Autodesk Fusion 360 part; units mm, degrees
(part 2 of 5)
  spline S13 degree 5 poles (-172.8984, -52.5106) (-172.8973, -52.5173) (-172.8952, -52.5307) (-172.8927, -52.5509) (-172.8903, -52.5779) (-172.8889, -52.6119) (-172.8884, -52.6459) (-172.8887, -52.6801) (-172.8892, -52.7143) (-172.89, -52.7486) (-172.8911, -52.7829) (-172.8924, -52.8172) (-172.8943, -52.8516) (-172.8966, -52.886) (-172.8994, -52.9205) (-172.9027, -52.955) (-172.9064, -52.9895) (-172.9104, -53.0241) (-172.9148, -53.0587) (-172.9194, -53.0933) (-172.9243, -53.1279) (-172.9295, -53.1625) (-172.9351, -53.1972) (-172.9409, -53.2319) (-172.9471, -53.2666) (-172.9535, -53.3013) (-172.9603, -53.336) (-172.9673, -53.3707) (-172.9746, -53.4054) (-172.9822, -53.4402) (-172.99, -53.4749) (-172.9981, -53.5097) (-173.0064, -53.5444) (-173.015, -53.5792) (-173.0239, -53.614) (-173.033, -53.6487) (-173.0424, -53.6835) (-173.052, -53.7183) (-173.0618, -53.753) (-173.0719, -53.7878) (-173.0822, -53.8225) (-173.0928, -53.8573) (-173.1036, -53.892) (-173.1146, -53.9267) (-173.1259, -53.9615) (-173.1373, -53.9962) (-173.1491, -54.0309) (-173.161, -54.0656) (-173.1731, -54.1003) (-173.1855, -54.135) (-173.1981, -54.1696) (-173.2109, -54.2043) (-173.2239, -54.2389) (-173.2371, -54.2735) (-173.2506, -54.3081) (-173.2642, -54.3427) (-173.2781, -54.3773) (-173.2921, -54.4118) (-173.3064, -54.4464) (-173.3209, -54.4809) (-173.3356, -54.5154) (-173.3504, -54.5499) (-173.3655, -54.5843) (-173.3808, -54.6188) (-173.3963, -54.6532) (-173.412, -54.6875) (-173.4278, -54.7219) (-173.4439, -54.7562) (-173.4602, -54.7906) (-173.4766, -54.8248) (-173.4933, -54.8591) (-173.5068, -54.8865) (-173.517, -54.907) (-173.5238, -54.9207) (-173.5272, -54.9275) knots 0 0 0 0 0 0 0.01428571 0.02857143 0.04285714 0.05714286 0.07142857 0.08571429 0.1 0.11428571 0.12857143 0.14285714 0.15714286 0.17142857 0.18571429 0.2 0.21428571 0.22857143 0.24285714 0.25714286 0.27142857 0.28571429 0.3 0.31428571 0.32857143 0.34285714 0.35714286 0.37142857 0.38571429 0.4 0.41428571 0.42857143 0.44285714 0.45714286 0.47142857 0.48571429 0.5 0.51428571 0.52857143 0.54285714 0.55714286 0.57142857 0.58571429 0.6 0.61428571 0.62857143 0.64285714 0.65714286 0.67142857 0.68571429 0.7 0.71428571 0.72857143 0.74285714 0.75714286 0.77142857 0.78571429 0.8 0.81428571 0.82857143 0.84285714 0.85714286 0.87142857 0.88571429 0.9 0.91428571 0.92857143 0.94285714 0.95714286 0.97142857 0.98571429 1 1 1 1 1 1
  line L13 (-172.8984, -52.5106) -> (-172.9699, -52.085)
  arc A26 (-172.5797, -51.5128) -> (-172.9699, -52.085) centre (-172.4768, -52.0021) ccw
  arc A27 (-172.5797, -51.5128) -> (-171.7948, -51.3195) centre (-175, -40) ccw
  arc A28 (-171.1835, -51.6448) -> (-171.7948, -51.3195) centre (-171.6586, -51.8006) ccw
  line L14 (-171.1835, -51.6448) -> (-171.0491, -52.0549)
  spline S14 degree 5 poles (-171.0491, -52.0549) (-171.047, -52.0614) (-171.0426, -52.0742) (-171.0354, -52.0933) (-171.025, -52.1183) (-171.0105, -52.1491) (-170.995, -52.1794) (-170.979, -52.2096) (-170.9626, -52.2396) (-170.9459, -52.2696) (-170.9291, -52.2995) (-170.9119, -52.3292) (-170.8943, -52.3588) (-170.8763, -52.3882) (-170.8578, -52.4175) (-170.8388, -52.4465) (-170.8195, -52.4753) (-170.7999, -52.5041) (-170.78, -52.5327) (-170.7598, -52.5612) (-170.7393, -52.5895) (-170.7186, -52.6178) (-170.6977, -52.6459) (-170.6764, -52.6739) (-170.6548, -52.7018) (-170.633, -52.7295) (-170.6109, -52.7571) (-170.5885, -52.7846) (-170.5659, -52.812) (-170.543, -52.8392) (-170.52, -52.8664) (-170.4967, -52.8934) (-170.4731, -52.9203) (-170.4494, -52.9471) (-170.4254, -52.9737) (-170.4011, -53.0003) (-170.3767, -53.0267) (-170.352, -53.053) (-170.3272, -53.0792) (-170.3021, -53.1053) (-170.2768, -53.1313) (-170.2513, -53.1572) (-170.2256, -53.1829) (-170.1997, -53.2086) (-170.1736, -53.2341) (-170.1473, -53.2595) (-170.1208, -53.2848) (-170.0942, -53.31) (-170.0673, -53.3351) (-170.0402, -53.36) (-170.013, -53.3849) (-169.9856, -53.4096) (-169.9579, -53.4342) (-169.9301, -53.4588) (-169.9022, -53.4832) (-169.874, -53.5074) (-169.8457, -53.5316) (-169.8172, -53.5557) (-169.7885, -53.5796) (-169.7596, -53.6035) (-169.7306, -53.6272) (-169.7014, -53.6508) (-169.6721, -53.6743) (-169.6425, -53.6977) (-169.6128, -53.721) (-169.583, -53.7442) (-169.553, -53.7672) (-169.5228, -53.7901) (-169.4924, -53.813) (-169.4619, -53.8357) (-169.4313, -53.8583) (-169.4066, -53.8763) (-169.388, -53.8897) (-169.3756, -53.8986) (-169.3694, -53.9031) knots 0 0 0 0 0 0 0.01428571 0.02857143 0.04285714 0.05714286 0.07142857 0.08571429 0.1 0.11428571 0.12857143 0.14285714 0.15714286 0.17142857 0.18571429 0.2 0.21428571 0.22857143 0.24285714 0.25714286 0.27142857 0.28571429 0.3 0.31428571 0.32857143 0.34285714 0.35714286 0.37142857 0.38571429 0.4 0.41428571 0.42857143 0.44285714 0.45714286 0.47142857 0.48571429 0.5 0.51428571 0.52857143 0.54285714 0.55714286 0.57142857 0.58571429 0.6 0.61428571 0.62857143 0.64285714 0.65714286 0.67142857 0.68571429 0.7 0.71428571 0.72857143 0.74285714 0.75714286 0.77142857 0.78571429 0.8 0.81428571 0.82857143 0.84285714 0.85714286 0.87142857 0.88571429 0.9 0.91428571 0.92857143 0.94285714 0.95714286 0.97142857 0.98571429 1 1 1 1 1 1
  arc A29 (-169.3694, -53.9031) -> (-168.5105, -53.5236) centre (-175, -40) ccw
  spline S15 degree 5 poles (-168.7463, -51.0373) (-168.7429, -51.0432) (-168.7364, -51.0551) (-168.7271, -51.0732) (-168.7157, -51.0978) (-168.7027, -51.1292) (-168.6906, -51.1611) (-168.6791, -51.1933) (-168.668, -51.2256) (-168.657, -51.2581) (-168.6463, -51.2907) (-168.6358, -51.3234) (-168.6257, -51.3563) (-168.6161, -51.3895) (-168.607, -51.4228) (-168.5983, -51.4564) (-168.59, -51.4901) (-168.582, -51.524) (-168.5742, -51.5579) (-168.5667, -51.592) (-168.5595, -51.6263) (-168.5526, -51.6606) (-168.5459, -51.695) (-168.5395, -51.7296) (-168.5334, -51.7643) (-168.5276, -51.7992) (-168.5221, -51.8341) (-168.5168, -51.8691) (-168.5118, -51.9043) (-168.507, -51.9395) (-168.5025, -51.9748) (-168.4982, -52.0103) (-168.4942, -52.0458) (-168.4904, -52.0814) (-168.4868, -52.1171) (-168.4835, -52.1529) (-168.4804, -52.1887) (-168.4775, -52.2247) (-168.4749, -52.2607) (-168.4725, -52.2968) (-168.4703, -52.333) (-168.4684, -52.3693) (-168.4666, -52.4056) (-168.4651, -52.442) (-168.4638, -52.4785) (-168.4627, -52.5151) (-168.4618, -52.5517) (-168.4612, -52.5884) (-168.4607, -52.6251) (-168.4605, -52.6619) (-168.4604, -52.6988) (-168.4606, -52.7357) (-168.461, -52.7727) (-168.4616, -52.8098) (-168.4624, -52.8469) (-168.4634, -52.8841) (-168.4646, -52.9213) (-168.466, -52.9586) (-168.4676, -52.9959) (-168.4694, -53.0333) (-168.4714, -53.0707) (-168.4736, -53.1082) (-168.476, -53.1458) (-168.4785, -53.1833) (-168.4813, -53.221) (-168.4843, -53.2586) (-168.4875, -53.2964) (-168.4908, -53.3341) (-168.4944, -53.3719) (-168.4981, -53.4098) (-168.5021, -53.4477) (-168.5053, -53.478) (-168.5079, -53.5008) (-168.5097, -53.516) (-168.5105, -53.5236) knots 0 0 0 0 0 0 0.01428571 0.02857143 0.04285714 0.05714286 0.07142857 0.08571429 0.1 0.11428571 0.12857143 0.14285714 0.15714286 0.17142857 0.18571429 0.2 0.21428571 0.22857143 0.24285714 0.25714286 0.27142857 0.28571429 0.3 0.31428571 0.32857143 0.34285714 0.35714286 0.37142857 0.38571429 0.4 0.41428571 0.42857143 0.44285714 0.45714286 0.47142857 0.48571429 0.5 0.51428571 0.52857143 0.54285714 0.55714286 0.57142857 0.58571429 0.6 0.61428571 0.62857143 0.64285714 0.65714286 0.67142857 0.68571429 0.7 0.71428571 0.72857143 0.74285714 0.75714286 0.77142857 0.78571429 0.8 0.81428571 0.82857143 0.84285714 0.85714286 0.87142857 0.88571429 0.9 0.91428571 0.92857143 0.94285714 0.95714286 0.97142857 0.98571429 1 1 1 1 1 1
  line L15 (-168.7463, -51.0373) -> (-168.959, -50.6618)
  arc A30 (-168.788, -49.9907) -> (-168.959, -50.6618) centre (-168.524, -50.4153) ccw
  arc A31 (-168.788, -49.9907) -> (-168.1167, -49.5406) centre (-175, -40) ccw
  arc A32 (-167.4309, -49.6372) -> (-168.1167, -49.5406) centre (-167.8241, -49.9461) ccw
  line L16 (-167.4309, -49.6372) -> (-167.1643, -49.9766)
  spline S16 degree 5 poles (-167.1643, -49.9766) (-167.1601, -49.982) (-167.1516, -49.9925) (-167.1384, -50.008) (-167.12, -50.0279) (-167.0959, -50.0519) (-167.0709, -50.0752) (-167.0455, -50.098) (-167.0199, -50.1206) (-166.994, -50.1431) (-166.9679, -50.1654) (-166.9416, -50.1875) (-166.915, -50.2093) (-166.888, -50.2308) (-166.8606, -50.2519) (-166.8329, -50.2727) (-166.8048, -50.2932) (-166.7765, -50.3134) (-166.748, -50.3335) (-166.7193, -50.3534) (-166.6904, -50.3731) (-166.6613, -50.3925) (-166.632, -50.4118) (-166.6024, -50.4308) (-166.5726, -50.4496) (-166.5426, -50.4682) (-166.5124, -50.4866) (-166.4819, -50.5048) (-166.4513, -50.5228) (-166.4206, -50.5406) (-166.3896, -50.5582) (-166.3585, -50.5756) (-166.3271, -50.5928) (-166.2956, -50.6099) (-166.264, -50.6267) (-166.2321, -50.6434) (-166.2001, -50.6599) (-166.1679, -50.6762) (-166.1356, -50.6923) (-166.1031, -50.7082) (-166.0705, -50.724) (-166.0377, -50.7396) (-166.0047, -50.755) (-165.9716, -50.7702) (-165.9384, -50.7853) (-165.905, -50.8001) (-165.8714, -50.8149) (-165.8377, -50.8294) (-165.8039, -50.8438) (-165.7699, -50.858) (-165.7358, -50.872) (-165.7016, -50.8859) (-165.6672, -50.8996) (-165.6327, -50.9131) (-165.5981, -50.9265) (-165.5633, -50.9397) (-165.5284, -50.9527) (-165.4934, -50.9655) (-165.4583, -50.9782) (-165.423, -50.9908) (-165.3876, -51.0031) (-165.3521, -51.0153) (-165.3165, -51.0274) (-165.2807, -51.0393) (-165.2449, -51.051) (-165.2089, -51.0625) (-165.1728, -51.0739) (-165.1366, -51.0852) (-165.1003, -51.0962) (-165.0638, -51.1072) (-165.0273, -51.1179) (-164.998, -51.1264) (-164.9759, -51.1327) (-164.9612, -51.1368) (-164.9538, -51.1389) knots 0 0 0 0 0 0 0.01428571 0.02857143 0.04285714 0.05714286 0.07142857 0.08571429 0.1 0.11428571 0.12857143 0.14285714 0.15714286 0.17142857 0.18571429 0.2 0.21428571 0.22857143 0.24285714 0.25714286 0.27142857 0.28571429 0.3 0.31428571 0.32857143 0.34285714 0.35714286 0.37142857 0.38571429 0.4 0.41428571 0.42857143 0.44285714 0.45714286 0.47142857 0.48571429 0.5 0.51428571 0.52857143 0.54285714 0.55714286 0.57142857 0.58571429 0.6 0.61428571 0.62857143 0.64285714 0.65714286 0.67142857 0.68571429 0.7 0.71428571 0.72857143 0.74285714 0.75714286 0.77142857 0.78571429 0.8 0.81428571 0.82857143 0.84285714 0.85714286 0.87142857 0.88571429 0.9 0.91428571 0.92857143 0.94285714 0.95714286 0.97142857 0.98571429 1 1 1 1 1 1
  arc A33 (-164.9538, -51.1389) -> (-164.2766, -50.4885) centre (-175, -40) ccw
  spline S17 degree 5 poles (-165.3485, -48.2328) (-165.3433, -48.2372) (-165.3331, -48.2461) (-165.3182, -48.26) (-165.299, -48.2792) (-165.276, -48.3042) (-165.2538, -48.3301) (-165.232, -48.3564) (-165.2104, -48.383) (-165.189, -48.4097) (-165.1678, -48.4367) (-165.1468, -48.4638) (-165.1261, -48.4913) (-165.1057, -48.5192) (-165.0857, -48.5474) (-165.0661, -48.576) (-165.0467, -48.6048) (-165.0276, -48.6339) (-165.0087, -48.6632) (-164.99, -48.6927) (-164.9715, -48.7223) (-164.9532, -48.7522) (-164.9352, -48.7823) (-164.9174, -48.8126) (-164.8998, -48.8432) (-164.8824, -48.8739) (-164.8653, -48.9048) (-164.8483, -48.936) (-164.8316, -48.9673) (-164.8151, -48.9987) (-164.7987, -49.0304) (-164.7826, -49.0622) (-164.7666, -49.0942) (-164.7509, -49.1264) (-164.7353, -49.1587) (-164.72, -49.1912) (-164.7048, -49.2238) (-164.6898, -49.2566) (-164.675, -49.2896) (-164.6604, -49.3227) (-164.646, -49.356) (-164.6317, -49.3894) (-164.6177, -49.4229) (-164.6038, -49.4566) (-164.5901, -49.4904) (-164.5765, -49.5244) (-164.5632, -49.5585) (-164.55, -49.5928) (-164.537, -49.6272) (-164.5242, -49.6617) (-164.5116, -49.6963) (-164.4991, -49.7311) (-164.4868, -49.766) (-164.4747, -49.801) (-164.4628, -49.8361) (-164.451, -49.8714) (-164.4394, -49.9068) (-164.4279, -49.9423) (-164.4167, -49.9779) (-164.4056, -50.0137) (-164.3946, -50.0495) (-164.3839, -50.0855) (-164.3733, -50.1216) (-164.3629, -50.1578) (-164.3526, -50.1941) (-164.3425, -50.2305) (-164.3326, -50.2671) (-164.3228, -50.3037) (-164.3132, -50.3404) (-164.3038, -50.3773) (-164.2946, -50.4142) (-164.2873, -50.4439) (-164.2819, -50.4662) (-164.2783, -50.481) (-164.2766, -50.4885) knots 0 0 0 0 0 0 0.01428571 0.02857143 0.04285714 0.05714286 0.07142857 0.08571429 0.1 0.11428571 0.12857143 0.14285714 0.15714286 0.17142857 0.18571429 0.2 0.21428571 0.22857143 0.24285714 0.25714286 0.27142857 0.28571429 0.3 0.31428571 0.32857143 0.34285714 0.35714286 0.37142857 0.38571429 0.4 0.41428571 0.42857143 0.44285714 0.45714286 0.47142857 0.48571429 0.5 0.51428571 0.52857143 0.54285714 0.55714286 0.57142857 0.58571429 0.6 0.61428571 0.62857143 0.64285714 0.65714286 0.67142857 0.68571429 0.7 0.71428571 0.72857143 0.74285714 0.75714286 0.77142857 0.78571429 0.8 0.81428571 0.82857143 0.84285714 0.85714286 0.87142857 0.88571429 0.9 0.91428571 0.92857143 0.94285714 0.95714286 0.97142857 0.98571429 1 1 1 1 1 1
  line L17 (-165.3485, -48.2328) -> (-165.6768, -47.9527)
  arc A34 (-165.7456, -47.2636) -> (-165.6768, -47.9527) centre (-165.3523, -47.5723) ccw
  arc A35 (-165.7456, -47.2636) -> (-165.2687, -46.611) centre (-175, -40) ccw
  arc A36 (-164.5912, -46.4673) -> (-165.2687, -46.611) centre (-164.8551, -46.892) ccw
  line L18 (-164.5912, -46.4673) -> (-164.2247, -46.695)
  spline S18 degree 5 poles (-164.2247, -46.695) (-164.2189, -46.6986) (-164.2073, -46.7056) (-164.1896, -46.7156) (-164.1654, -46.728) (-164.1346, -46.7423) (-164.1032, -46.7557) (-164.0715, -46.7684) (-164.0397, -46.7809) (-164.0077, -46.7932) (-163.9755, -46.8052) (-163.9433, -46.817) (-163.9108, -46.8284) (-163.8781, -46.8393) (-163.8451, -46.8498) (-163.8119, -46.8598) (-163.7786, -46.8695) (-163.7451, -46.8789) (-163.7114, -46.888) (-163.6776, -46.8969) (-163.6437, -46.9055) (-163.6097, -46.9138) (-163.5756, -46.9219) (-163.5413, -46.9296) (-163.5068, -46.9371) (-163.4723, -46.9443) (-163.4376, -46.9512) (-163.4028, -46.9579) (-163.3679, -46.9644) (-163.3329, -46.9705) (-163.2978, -46.9765) (-163.2625, -46.9822) (-163.2272, -46.9877) (-163.1918, -46.9929) (-163.1563, -46.9979) (-163.1207, -47.0027) (-163.0849, -47.0073) (-163.0491, -47.0116) (-163.0132, -47.0156) (-162.9772, -47.0195) (-162.9412, -47.0232) (-162.905, -47.0266) (-162.8688, -47.0298) (-162.8325, -47.0328) (-162.7961, -47.0356) (-162.7596, -47.0381) (-162.723, -47.0405) (-162.6864, -47.0426) (-162.6497, -47.0446) (-162.6129, -47.0463) (-162.5761, -47.0478) (-162.5392, -47.0491) (-162.5022, -47.0503) (-162.4651, -47.0512) (-162.428, -47.0519) (-162.3909, -47.0524) (-162.3536, -47.0527) (-162.3163, -47.0528) (-162.2789, -47.0527) (-162.2415, -47.0524) (-162.204, -47.0519) (-162.1665, -47.0513) (-162.1289, -47.0504) (-162.0912, -47.0493) (-162.0535, -47.0481) (-162.0157, -47.0466) (-161.9779, -47.045) (-161.9401, -47.0432) (-161.9021, -47.0411) (-161.8642, -47.0389) (-161.8262, -47.0365) (-161.7957, -47.0345) (-161.7729, -47.0328) (-161.7576, -47.0317) (-161.75, -47.0311) knots 0 0 0 0 0 0 0.01428571 0.02857143 0.04285714 0.05714286 0.07142857 0.08571429 0.1 0.11428571 0.12857143 0.14285714 0.15714286 0.17142857 0.18571429 0.2 0.21428571 0.22857143 0.24285714 0.25714286 0.27142857 0.28571429 0.3 0.31428571 0.32857143 0.34285714 0.35714286 0.37142857 0.38571429 0.4 0.41428571 0.42857143 0.44285714 0.45714286 0.47142857 0.48571429 0.5 0.51428571 0.52857143 0.54285714 0.55714286 0.57142857 0.58571429 0.6 0.61428571 0.62857143 0.64285714 0.65714286 0.67142857 0.68571429 0.7 0.71428571 0.72857143 0.74285714 0.75714286 0.77142857 0.78571429 0.8 0.81428571 0.82857143 0.84285714 0.85714286 0.87142857 0.88571429 0.9 0.91428571 0.92857143 0.94285714 0.95714286 0.97142857 0.98571429 1 1 1 1 1 1
  arc A37 (-161.75, -47.0311) -> (-161.336, -46.1883) centre (-175, -40) ccw
  spline S19 degree 5 poles (-163.1147, -44.4353) (-163.1084, -44.4376) (-163.0957, -44.4425) (-163.077, -44.4504) (-163.0524, -44.4619) (-163.0222, -44.4776) (-162.9925, -44.4943) (-162.963, -44.5116) (-162.9337, -44.5292) (-162.9044, -44.547) (-162.8752, -44.5651) (-162.8462, -44.5834) (-162.8173, -44.6022) (-162.7887, -44.6214) (-162.7602, -44.6411) (-162.732, -44.6612) (-162.704, -44.6816) (-162.676, -44.7024) (-162.6483, -44.7235) (-162.6206, -44.7448) (-162.5931, -44.7664) (-162.5657, -44.7882) (-162.5384, -44.8103) (-162.5113, -44.8327) (-162.4844, -44.8554) (-162.4575, -44.8783) (-162.4308, -44.9015) (-162.4043, -44.925) (-162.3778, -44.9487) (-162.3515, -44.9726) (-162.3254, -44.9968) (-162.2993, -45.0211) (-162.2734, -45.0457) (-162.2476, -45.0706) (-162.2219, -45.0956) (-162.1964, -45.1209) (-162.1709, -45.1464) (-162.1456, -45.1721) (-162.1205, -45.198) (-162.0954, -45.2241) (-162.0705, -45.2504) (-162.0457, -45.277) (-162.021, -45.3037) (-161.9964, -45.3306) (-161.9719, -45.3577) (-161.9476, -45.385) (-161.9234, -45.4125) (-161.8993, -45.4402) (-161.8754, -45.468) (-161.8515, -45.4961) (-161.8278, -45.5243) (-161.8042, -45.5527) (-161.7807, -45.5813) (-161.7573, -45.6101) (-161.7341, -45.639) (-161.7109, -45.6681) (-161.6879, -45.6974) (-161.665, -45.7269) (-161.6423, -45.7565) (-161.6196, -45.7863) (-161.5971, -45.8162) (-161.5747, -45.8464) (-161.5524, -45.8767) (-161.5302, -45.9071) (-161.5081, -45.9377) (-161.4862, -45.9685) (-161.4644, -45.9994) (-161.4427, -46.0305) (-161.4211, -46.0618) (-161.3996, -46.0931) (-161.3783, -46.1247) (-161.3613, -46.1501) (-161.3486, -46.1692) (-161.3402, -46.1819) (-161.336, -46.1883) knots 0 0 0 0 0 0 0.01428571 0.02857143 0.04285714 0.05714286 0.07142857 0.08571429 0.1 0.11428571 0.12857143 0.14285714 0.15714286 0.17142857 0.18571429 0.2 0.21428571 0.22857143 0.24285714 0.25714286 0.27142857 0.28571429 0.3 0.31428571 0.32857143 0.34285714 0.35714286 0.37142857 0.38571429 0.4 0.41428571 0.42857143 0.44285714 0.45714286 0.47142857 0.48571429 0.5 0.51428571 0.52857143 0.54285714 0.55714286 0.57142857 0.58571429 0.6 0.61428571 0.62857143 0.64285714 0.65714286 0.67142857 0.68571429 0.7 0.71428571 0.72857143 0.74285714 0.75714286 0.77142857 0.78571429 0.8 0.81428571 0.82857143 0.84285714 0.85714286 0.87142857 0.88571429 0.9 0.91428571 0.92857143 0.94285714 0.95714286 0.97142857 0.98571429 1 1 1 1 1 1
  line L19 (-163.1147, -44.4353) -> (-163.5191, -44.2844)
  arc A38 (-163.8194, -43.6604) -> (-163.5191, -44.2844) centre (-163.3442, -43.8159) ccw
  arc A39 (-163.8194, -43.6604) -> (-163.5945, -42.884) centre (-175, -40) ccw
  arc A40 (-163.007, -42.5172) -> (-163.5945, -42.884) centre (-163.1097, -43.0066) ccw
  line L20 (-163.007, -42.5172) -> (-162.5847, -42.6059)
  spline S20 degree 5 poles (-162.5847, -42.6059) (-162.578, -42.6073) (-162.5647, -42.6099) (-162.5446, -42.6132) (-162.5177, -42.6167) (-162.4838, -42.6195) (-162.4498, -42.6213) (-162.4157, -42.6225) (-162.3814, -42.6233) (-162.3472, -42.6239) (-162.3129, -42.6242) (-162.2785, -42.6242) (-162.2441, -42.6238) (-162.2096, -42.6229) (-162.1751, -42.6215) (-162.1405, -42.6196) (-162.1058, -42.6173) (-162.0711, -42.6146) (-162.0364, -42.6117) (-162.0016, -42.6084) (-161.9668, -42.6049) (-161.932, -42.6011) (-161.8971, -42.597) (-161.8622, -42.5926) (-161.8273, -42.5879) (-161.7924, -42.5828) (-161.7574, -42.5774) (-161.7224, -42.5718) (-161.6874, -42.5659) (-161.6524, -42.5598) (-161.6174, -42.5534) (-161.5823, -42.5467) (-161.5473, -42.5398) (-161.5122, -42.5326) (-161.4771, -42.5251) (-161.442, -42.5174) (-161.4069, -42.5095) (-161.3718, -42.5013) (-161.3366, -42.4928) (-161.3015, -42.4842) (-161.2664, -42.4753) (-161.2312, -42.4661) (-161.1961, -42.4567) (-161.1609, -42.4471) (-161.1258, -42.4373) (-161.0906, -42.4272) (-161.0554, -42.4169) (-161.0203, -42.4064) (-160.9851, -42.3957) (-160.95, -42.3847) (-160.9149, -42.3736) (-160.8797, -42.3622) (-160.8446, -42.3506) (-160.8095, -42.3388) (-160.7743, -42.3267) (-160.7392, -42.3145) (-160.7041, -42.302) (-160.669, -42.2894) (-160.6339, -42.2765) (-160.5989, -42.2635) (-160.5638, -42.2502) (-160.5288, -42.2367) (-160.4937, -42.223) (-160.4587, -42.2091) (-160.4237, -42.1951) (-160.3887, -42.1808) (-160.3537, -42.1663) (-160.3188, -42.1516) (-160.2838, -42.1368) (-160.2489, -42.1217) (-160.214, -42.1065) (-160.1861, -42.0941) (-160.1652, -42.0848) (-160.1512, -42.0785) (-160.1443, -42.0753) knots 0 0 0 0 0 0 0.01428571 0.02857143 0.04285714 0.05714286 0.07142857 0.08571429 0.1 0.11428571 0.12857143 0.14285714 0.15714286 0.17142857 0.18571429 0.2 0.21428571 0.22857143 0.24285714 0.25714286 0.27142857 0.28571429 0.3 0.31428571 0.32857143 0.34285714 0.35714286 0.37142857 0.38571429 0.4 0.41428571 0.42857143 0.44285714 0.45714286 0.47142857 0.48571429 0.5 0.51428571 0.52857143 0.54285714 0.55714286 0.57142857 0.58571429 0.6 0.61428571 0.62857143 0.64285714 0.65714286 0.67142857 0.68571429 0.7 0.71428571 0.72857143 0.74285714 0.75714286 0.77142857 0.78571429 0.8 0.81428571 0.82857143 0.84285714 0.85714286 0.87142857 0.88571429 0.9 0.91428571 0.92857143 0.94285714 0.95714286 0.97142857 0.98571429 1 1 1 1 1 1
  arc A41 (-160.1443, -42.0753) -> (-160.0435, -41.1417) centre (-175, -40) ccw
  spline S21 degree 5 poles (-162.3146, -40.1028) (-162.3078, -40.1028) (-162.2942, -40.1031) (-162.2739, -40.1041) (-162.2468, -40.1065) (-162.2131, -40.111) (-162.1795, -40.1165) (-162.1459, -40.1226) (-162.1123, -40.1291) (-162.0787, -40.1358) (-162.0451, -40.1428) (-162.0115, -40.1502) (-161.978, -40.1579) (-161.9445, -40.1662) (-161.9111, -40.1749) (-161.8777, -40.1842) (-161.8443, -40.1938) (-161.8109, -40.2038) (-161.7776, -40.2141) (-161.7444, -40.2247) (-161.7111, -40.2355) (-161.6779, -40.2466) (-161.6447, -40.2581) (-161.6116, -40.2699) (-161.5785, -40.282) (-161.5454, -40.2943) (-161.5124, -40.307) (-161.4795, -40.32) (-161.4465, -40.3332) (-161.4136, -40.3467) (-161.3807, -40.3604) (-161.3479, -40.3744) (-161.3151, -40.3887) (-161.2824, -40.4032) (-161.2497, -40.418) (-161.2171, -40.433) (-161.1844, -40.4482) (-161.1519, -40.4637) (-161.1194, -40.4795) (-161.0869, -40.4954) (-161.0545, -40.5116) (-161.0221, -40.5281) (-160.9897, -40.5447) (-160.9574, -40.5616) (-160.9252, -40.5787) (-160.893, -40.5961) (-160.8608, -40.6136) (-160.8287, -40.6314) (-160.7967, -40.6494) (-160.7647, -40.6676) (-160.7327, -40.686) (-160.7008, -40.7046) (-160.669, -40.7234) (-160.6372, -40.7425) (-160.6055, -40.7617) (-160.5738, -40.7812) (-160.5421, -40.8008) (-160.5105, -40.8207) (-160.479, -40.8407) (-160.4475, -40.861) (-160.4161, -40.8814) (-160.3847, -40.9021) (-160.3534, -40.9229) (-160.3222, -40.9439) (-160.291, -40.9651) (-160.2598, -40.9866) (-160.2287, -41.0082) (-160.1977, -41.0299) (-160.1668, -41.0519) (-160.1359, -41.0741) (-160.105, -41.0964) (-160.0804, -41.1145) (-160.0619, -41.1281) (-160.0497, -41.1372) (-160.0435, -41.1417) knots 0 0 0 0 0 0 0.01428571 0.02857143 0.04285714 0.05714286 0.07142857 0.08571429 0.1 0.11428571 0.12857143 0.14285714 0.15714286 0.17142857 0.18571429 0.2 0.21428571 0.22857143 0.24285714 0.25714286 0.27142857 0.28571429 0.3 0.31428571 0.32857143 0.34285714 0.35714286 0.37142857 0.38571429 0.4 0.41428571 0.42857143 0.44285714 0.45714286 0.47142857 0.48571429 0.5 0.51428571 0.52857143 0.54285714 0.55714286 0.57142857 0.58571429 0.6 0.61428571 0.62857143 0.64285714 0.65714286 0.67142857 0.68571429 0.7 0.71428571 0.72857143 0.74285714 0.75714286 0.77142857 0.78571429 0.8 0.81428571 0.82857143 0.84285714 0.85714286 0.87142857 0.88571429 0.9 0.91428571 0.92857143 0.94285714 0.95714286 0.97142857 0.98571429 1 1 1 1 1 1
  line L21 (-162.3146, -40.1028) -> (-162.7461, -40.0993)
  arc A42 (-163.2418, -39.6156) -> (-162.7461, -40.0993) centre (-162.742, -39.5993) ccw
  arc A43 (-163.2418, -39.6156) -> (-163.2959, -38.8091) centre (-175, -40) ccw
  arc A44 (-162.8693, -38.2636) -> (-163.2959, -38.8091) centre (-162.7985, -38.7585) ccw
  line L22 (-162.8693, -38.2636) -> (-162.4422, -38.2024)
  spline S22 degree 5 poles (-162.4422, -38.2024) (-162.4354, -38.2015) (-162.422, -38.1994) (-162.402, -38.1956) (-162.3755, -38.1897) (-162.3427, -38.1808) (-162.3101, -38.1708) (-162.2776, -38.1602) (-162.2452, -38.1493) (-162.2128, -38.1381) (-162.1805, -38.1267) (-162.1482, -38.115) (-162.116, -38.1028) (-162.0839, -38.0902) (-162.0519, -38.077) (-162.02, -38.0634) (-161.9883, -38.0494) (-161.9566, -38.035) (-161.9249, -38.0203) (-161.8934, -38.0054) (-161.8619, -37.9902) (-161.8304, -37.9747) (-161.7991, -37.959) (-161.7678, -37.9429) (-161.7366, -37.9265) (-161.7055, -37.9098) (-161.6745, -37.8928) (-161.6436, -37.8755) (-161.6127, -37.858) (-161.5819, -37.8403) (-161.5512, -37.8223) (-161.5205, -37.804) (-161.4899, -37.7855) (-161.4594, -37.7667) (-161.429, -37.7477) (-161.3986, -37.7285) (-161.3684, -37.709) (-161.3382, -37.6893) (-161.308, -37.6694) (-161.278, -37.6492) (-161.248, -37.6288) (-161.2181, -37.6082) (-161.1883, -37.5873) (-161.1585, -37.5663) (-161.1289, -37.545) (-161.0993, -37.5235) (-161.0698, -37.5019) (-161.0403, -37.48) (-161.011, -37.4578) (-160.9817, -37.4355) (-160.9525, -37.413) (-160.9234, -37.3903) (-160.8943, -37.3674) (-160.8653, -37.3443) (-160.8365, -37.3209) (-160.8077, -37.2974) (-160.7789, -37.2737) (-160.7503, -37.2498) (-160.7217, -37.2257) (-160.6932, -37.2015) (-160.6648, -37.177) (-160.6365, -37.1524) (-160.6082, -37.1275) (-160.5801, -37.1025) (-160.552, -37.0773) (-160.524, -37.0519) (-160.4961, -37.0264) (-160.4683, -37.0006) (-160.4405, -36.9747) (-160.4128, -36.9486) (-160.3853, -36.9223) (-160.3633, -36.9012) (-160.3468, -36.8852) (-160.3358, -36.8746) (-160.3304, -36.8692) knots 0 0 0 0 0 0 0.01428571 0.02857143 0.04285714 0.05714286 0.07142857 0.08571429 0.1 0.11428571 0.12857143 0.14285714 0.15714286 0.17142857 0.18571429 0.2 0.21428571 0.22857143 0.24285714 0.25714286 0.27142857 0.28571429 0.3 0.31428571 0.32857143 0.34285714 0.35714286 0.37142857 0.38571429 0.4 0.41428571 0.42857143 0.44285714 0.45714286 0.47142857 0.48571429 0.5 0.51428571 0.52857143 0.54285714 0.55714286 0.57142857 0.58571429 0.6 0.61428571 0.62857143 0.64285714 0.65714286 0.67142857 0.68571429 0.7 0.71428571 0.72857143 0.74285714 0.75714286 0.77142857 0.78571429 0.8 0.81428571 0.82857143 0.84285714 0.85714286 0.87142857 0.88571429 0.9 0.91428571 0.92857143 0.94285714 0.95714286 0.97142857 0.98571429 1 1 1 1 1 1
  arc A45 (-160.3304, -36.8692) -> (-160.555, -35.9575) centre (-175, -40) ccw
  spline S23 degree 5 poles (-163.0444, -35.7579) (-163.038, -35.7556) (-163.0252, -35.7513) (-163.0057, -35.7453) (-162.9795, -35.7383) (-162.9463, -35.7309) (-162.9128, -35.7246) (-162.8792, -35.7188) (-162.8454, -35.7135) (-162.8115, -35.7083) (-162.7775, -35.7034) (-162.7435, -35.6988) (-162.7093, -35.6946) (-162.675, -35.6909) (-162.6406, -35.6877) (-162.606, -35.6849) (-162.5714, -35.6826) (-162.5366, -35.6806) (-162.5018, -35.6789) (-162.4669, -35.6774) (-162.432, -35.6762) (-162.397, -35.6753) (-162.3619, -35.6748) (-162.3267, -35.6745) (-162.2915, -35.6745) (-162.2562, -35.6749) (-162.2208, -35.6755) (-162.1854, -35.6764) (-162.1499, -35.6775) (-162.1144, -35.679) (-162.0788, -35.6806) (-162.0432, -35.6826) (-162.0075, -35.6847) (-161.9718, -35.6872) (-161.936, -35.6899) (-161.9002, -35.6928) (-161.8643, -35.696) (-161.8284, -35.6994) (-161.7925, -35.7031) (-161.7565, -35.707) (-161.7205, -35.7111) (-161.6844, -35.7155) (-161.6483, -35.7201) (-161.6122, -35.7249) (-161.5761, -35.73) (-161.5399, -35.7352) (-161.5037, -35.7407) (-161.4674, -35.7465) (-161.4312, -35.7524) (-161.3949, -35.7585) (-161.3585, -35.7649) (-161.3222, -35.7715) (-161.2858, -35.7783) (-161.2494, -35.7853) (-161.213, -35.7925) (-161.1766, -35.8) (-161.1401, -35.8076) (-161.1037, -35.8155) (-161.0672, -35.8235) (-161.0307, -35.8318) (-160.9942, -35.8403) (-160.9576, -35.8489) (-160.9211, -35.8578) (-160.8845, -35.8669) (-160.8479, -35.8762) (-160.8114, -35.8856) (-160.7748, -35.8953) (-160.7382, -35.9052) (-160.7015, -35.9152) (-160.6649, -35.9255) (-160.6283, -35.9359) (-160.599, -35.9444) (-160.577, -35.9509) (-160.5623, -35.9553) (-160.555, -35.9575) knots 0 0 0 0 0 0 0.01428571 0.02857143 0.04285714 0.05714286 0.07142857 0.08571429 0.1 0.11428571 0.12857143 0.14285714 0.15714286 0.17142857 0.18571429 0.2 0.21428571 0.22857143 0.24285714 0.25714286 0.27142857 0.28571429 0.3 0.31428571 0.32857143 0.34285714 0.35714286 0.37142857 0.38571429 0.4 0.41428571 0.42857143 0.44285714 0.45714286 0.47142857 0.48571429 0.5 0.51428571 0.52857143 0.54285714 0.55714286 0.57142857 0.58571429 0.6 0.61428571 0.62857143 0.64285714 0.65714286 0.67142857 0.68571429 0.7 0.71428571 0.72857143 0.74285714 0.75714286 0.77142857 0.78571429 0.8 0.81428571 0.82857143 0.84285714 0.85714286 0.87142857 0.88571429 0.9 0.91428571 0.92857143 0.94285714 0.95714286 0.97142857 0.98571429 1 1 1 1 1 1
  line L23 (-163.0444, -35.7579) -> (-163.4511, -35.9022)
  arc A46 (-164.0823, -35.6173) -> (-163.4511, -35.9022) centre (-163.6183, -35.431) ccw
  arc A47 (-164.0823, -35.6173) -> (-164.4091, -34.8779) centre (-175, -40) ccw
  arc A48 (-164.1948, -34.2194) -> (-164.4091, -34.8779) centre (-163.9589, -34.6602) ccw
  line L24 (-164.1948, -34.2194) -> (-163.8143, -34.0158)
  spline S24 degree 5 poles (-163.8143, -34.0158) (-163.8083, -34.0126) (-163.7964, -34.006) (-163.7789, -33.9957) (-163.7561, -33.981) (-163.7283, -33.9614) (-163.701, -33.9409) (-163.6741, -33.9199) (-163.6474, -33.8985) (-163.6208, -33.8769) (-163.5943, -33.8551) (-163.568, -33.8331) (-163.5419, -33.8106) (-163.516, -33.7878) (-163.4905, -33.7645) (-163.4652, -33.7408) (-163.4401, -33.7167) (-163.4152, -33.6924) (-163.3905, -33.6678) (-163.366, -33.643) (-163.3416, -33.6179) (-163.3173, -33.5926) (-163.2933, -33.5671) (-163.2694, -33.5413) (-163.2457, -33.5152) (-163.2222, -33.4889) (-163.1989, -33.4623) (-163.1757, -33.4355) (-163.1526, -33.4085) (-163.1298, -33.3813) (-163.1071, -33.3538) (-163.0845, -33.3262) (-163.0621, -33.2983) (-163.0398, -33.2703) (-163.0177, -33.242) (-162.9958, -33.2135) (-162.974, -33.1849) (-162.9524, -33.156) (-162.9309, -33.127) (-162.9095, -33.0977) (-162.8884, -33.0683) (-162.8673, -33.0387) (-162.8464, -33.009) (-162.8257, -32.979) (-162.8051, -32.9489) (-162.7846, -32.9186) (-162.7643, -32.8881) (-162.7441, -32.8574) (-162.7241, -32.8266) (-162.7042, -32.7956) (-162.6845, -32.7645) (-162.6649, -32.7332) (-162.6454, -32.7017) (-162.6261, -32.6701) (-162.6069, -32.6383) (-162.5879, -32.6063) (-162.569, -32.5742) (-162.5502, -32.542) (-162.5316, -32.5096) (-162.5132, -32.477) (-162.4948, -32.4443) (-162.4767, -32.4115) (-162.4586, -32.3785) (-162.4407, -32.3453) (-162.4229, -32.3121) (-162.4053, -32.2786) (-162.3878, -32.2451) (-162.3705, -32.2113) (-162.3533, -32.1775) (-162.3362, -32.1435) (-162.3193, -32.1094) (-162.3058, -32.082) (-162.2958, -32.0614) (-162.2892, -32.0476) (-162.2858, -32.0407) knots 0 0 0 0 0 0 0.01428571 0.02857143 0.04285714 0.05714286 0.07142857 0.08571429 0.1 0.11428571 0.12857143 0.14285714 0.15714286 0.17142857 0.18571429 0.2 0.21428571 0.22857143 0.24285714 0.25714286 0.27142857 0.28571429 0.3 0.31428571 0.32857143 0.34285714 0.35714286 0.37142857 0.38571429 0.4 0.41428571 0.42857143 0.44285714 0.45714286 0.47142857 0.48571429 0.5 0.51428571 0.52857143 0.54285714 0.55714286 0.57142857 0.58571429 0.6 0.61428571 0.62857143 0.64285714 0.65714286 0.67142857 0.68571429 0.7 0.71428571 0.72857143 0.74285714 0.75714286 0.77142857 0.78571429 0.8 0.81428571 0.82857143 0.84285714 0.85714286 0.87142857 0.88571429 0.9 0.91428571 0.92857143 0.94285714 0.95714286 0.97142857 0.98571429 1 1 1 1 1 1
  arc A49 (-162.2858, -32.0407) -> (-162.8088, -31.2608) centre (-175, -40) ccw
  spline S25 degree 5 poles (-165.2163, -31.9247) (-165.2111, -31.9204) (-165.2005, -31.9119) (-165.1843, -31.8996) (-165.162, -31.884) (-165.1334, -31.8658) (-165.1041, -31.8484) (-165.0744, -31.8315) (-165.0445, -31.8148) (-165.0144, -31.7984) (-164.9842, -31.7822) (-164.9537, -31.7662) (-164.9231, -31.7506) (-164.8921, -31.7354) (-164.8609, -31.7206) (-164.8293, -31.7062) (-164.7976, -31.6921) (-164.7656, -31.6784) (-164.7335, -31.6648) (-164.7012, -31.6515) (-164.6687, -31.6385) (-164.6361, -31.6257) (-164.6034, -31.6131) (-164.5704, -31.6008) (-164.5373, -31.5888) (-164.504, -31.5771) (-164.4706, -31.5656) (-164.437, -31.5543) (-164.4032, -31.5432) (-164.3694, -31.5324) (-164.3354, -31.5218) (-164.3012, -31.5114) (-164.267, -31.5013) (-164.2325, -31.4914) (-164.198, -31.4817) (-164.1633, -31.4722) (-164.1286, -31.4629) (-164.0936, -31.4538) (-164.0586, -31.445) (-164.0235, -31.4363) (-163.9882, -31.4279) (-163.9528, -31.4197) (-163.9174, -31.4117) (-163.8818, -31.4038) (-163.8461, -31.3962) (-163.8103, -31.3888) (-163.7744, -31.3816) (-163.7383, -31.3746) (-163.7022, -31.3677) (-163.666, -31.3611) (-163.6297, -31.3547) (-163.5933, -31.3484) (-163.5568, -31.3424) (-163.5202, -31.3365) (-163.4835, -31.3309) (-163.4467, -31.3254) (-163.4099, -31.3201) (-163.3729, -31.315) (-163.3359, -31.3101) (-163.2987, -31.3054) (-163.2615, -31.3008) (-163.2242, -31.2965) (-163.1869, -31.2923) (-163.1494, -31.2884) (-163.1119, -31.2846) (-163.0742, -31.2809) (-163.0365, -31.2775) (-162.9988, -31.2743) (-162.9609, -31.2712) (-162.923, -31.2683) (-162.885, -31.2656) (-162.8545, -31.2636) (-162.8317, -31.2622) (-162.8164, -31.2612) (-162.8088, -31.2608) knots 0 0 0 0 0 0 0.01428571 0.02857143 0.04285714 0.05714286 0.07142857 0.08571429 0.1 0.11428571 0.12857143 0.14285714 0.15714286 0.17142857 0.18571429 0.2 0.21428571 0.22857143 0.24285714 0.25714286 0.27142857 0.28571429 0.3 0.31428571 0.32857143 0.34285714 0.35714286 0.37142857 0.38571429 0.4 0.41428571 0.42857143 0.44285714 0.45714286 0.47142857 0.48571429 0.5 0.51428571 0.52857143 0.54285714 0.55714286 0.57142857 0.58571429 0.6 0.61428571 0.62857143 0.64285714 0.65714286 0.67142857 0.68571429 0.7 0.71428571 0.72857143 0.74285714 0.75714286 0.77142857 0.78571429 0.8 0.81428571 0.82857143 0.84285714 0.85714286 0.87142857 0.88571429 0.9 0.91428571 0.92857143 0.94285714 0.95714286 0.97142857 0.98571429 1 1 1 1 1 1
  line L25 (-165.2163, -31.9247) -> (-165.5491, -32.1994)
  arc A50 (-166.2397, -32.1475) -> (-165.5491, -32.1994) centre (-165.8674, -31.8138) ccw
  arc A51 (-166.2397, -32.1475) -> (-166.7996, -31.5645) centre (-175, -40) ccw
  arc A52 (-166.8235, -30.8724) -> (-166.7996, -31.5645) centre (-166.4511, -31.206) ccw
  line L26 (-166.8235, -30.8724) -> (-166.5356, -30.5509)
  spline S26 degree 5 poles (-166.5356, -30.5509) (-166.5311, -30.5459) (-166.5221, -30.5357) (-166.5092, -30.52) (-166.4928, -30.4984) (-166.4734, -30.4704) (-166.4548, -30.4419) (-166.4367, -30.4129) (-166.4189, -30.3837) (-166.4012, -30.3543) (-166.3838, -30.3247) (-166.3666, -30.295) (-166.3498, -30.265) (-166.3333, -30.2347) (-166.3173, -30.204) (-166.3016, -30.1731) (-166.2863, -30.1419) (-166.2712, -30.1106) (-166.2564, -30.079) (-166.2418, -30.0473) (-166.2275, -30.0154) (-166.2133, -29.9833) (-166.1995, -29.9511) (-166.1859, -29.9187) (-166.1725, -29.8861) (-166.1594, -29.8533) (-166.1466, -29.8203) (-166.134, -29.7872) (-166.1216, -29.754) (-166.1094, -29.7206) (-166.0974, -29.687) (-166.0857, -29.6533) (-166.0741, -29.6195) (-166.0628, -29.5855) (-166.0517, -29.5514) (-166.0408, -29.5171) (-166.0302, -29.4827) (-166.0197, -29.4482) (-166.0095, -29.4136) (-165.9994, -29.3788) (-165.9895, -29.3439) (-165.9799, -29.3089) (-165.9704, -29.2738) (-165.9612, -29.2386) (-165.9521, -29.2032) (-165.9433, -29.1677) (-165.9346, -29.1321) (-165.9261, -29.0964) (-165.9178, -29.0606) (-165.9098, -29.0247) (-165.9019, -28.9887) (-165.8942, -28.9526) (-165.8866, -28.9163) (-165.8793, -28.88) (-165.8722, -28.8436) (-165.8652, -28.807) (-165.8584, -28.7704) (-165.8518, -28.7337) (-165.8454, -28.6969) (-165.8392, -28.66) (-165.8332, -28.623) (-165.8273, -28.5859) (-165.8217, -28.5487) (-165.8162, -28.5114) (-165.8109, -28.4741) (-165.8057, -28.4366) (-165.8008, -28.3991) (-165.796, -28.3615) (-165.7914, -28.3238) (-165.787, -28.286) (-165.7827, -28.2482) (-165.7795, -28.2178) (-165.7771, -28.195) (-165.7756, -28.1798) (-165.7748, -28.1722) knots 0 0 0 0 0 0 0.01428571 0.02857143 0.04285714 0.05714286 0.07142857 0.08571429 0.1 0.11428571 0.12857143 0.14285714 0.15714286 0.17142857 0.18571429 0.2 0.21428571 0.22857143 0.24285714 0.25714286 0.27142857 0.28571429 0.3 0.31428571 0.32857143 0.34285714 0.35714286 0.37142857 0.38571429 0.4 0.41428571 0.42857143 0.44285714 0.45714286 0.47142857 0.48571429 0.5 0.51428571 0.52857143 0.54285714 0.55714286 0.57142857 0.58571429 0.6 0.61428571 0.62857143 0.64285714 0.65714286 0.67142857 0.68571429 0.7 0.71428571 0.72857143 0.74285714 0.75714286 0.77142857 0.78571429 0.8 0.81428571 0.82857143 0.84285714 0.85714286 0.87142857 0.88571429 0.9 0.91428571 0.92857143 0.94285714 0.95714286 0.97142857 0.98571429 1 1 1 1 1 1
  arc A53 (-165.7748, -28.1722) -> (-166.533, -27.6182) centre (-175, -40) ccw
  spline S27 degree 5 poles (-168.5683, -29.0655) (-168.5648, -29.0596) (-168.5578, -29.048) (-168.5468, -29.0309) (-168.5312, -29.0087) (-168.5105, -28.9817) (-168.4889, -28.9554) (-168.4668, -28.9293) (-168.4443, -28.9035) (-168.4217, -28.8777) (-168.3989, -28.8522) (-168.3757, -28.8267) (-168.3523, -28.8016) (-168.3284, -28.7767) (-168.304, -28.7521) (-168.2793, -28.7278) (-168.2543, -28.7037) (-168.229, -28.6798) (-168.2034, -28.6561) (-168.1776, -28.6326) (-168.1516, -28.6092) (-168.1254, -28.5861) (-168.0989, -28.563) (-168.0721, -28.5402) (-168.0451, -28.5176) (-168.0178, -28.4952) (-167.9903, -28.4729) (-167.9626, -28.4509) (-167.9347, -28.4289) (-167.9066, -28.4072) (-167.8782, -28.3856) (-167.8497, -28.3642) (-167.821, -28.3429) (-167.792, -28.3218) (-167.7629, -28.3009) (-167.7336, -28.2801) (-167.704, -28.2595) (-167.6743, -28.239) (-167.6445, -28.2187) (-167.6144, -28.1986) (-167.5841, -28.1786) (-167.5537, -28.1588) (-167.5231, -28.1391) (-167.4923, -28.1196) (-167.4614, -28.1002) (-167.4303, -28.081) (-167.399, -28.0619) (-167.3676, -28.043) (-167.336, -28.0243) (-167.3042, -28.0056) (-167.2723, -27.9872) (-167.2402, -27.9689) (-167.208, -27.9507) (-167.1756, -27.9327) (-167.1431, -27.9148) (-167.1104, -27.8971) (-167.0775, -27.8795) (-167.0446, -27.8621) (-167.0114, -27.8448) (-166.9781, -27.8277) (-166.9447, -27.8107) (-166.9112, -27.7938) (-166.8775, -27.7771) (-166.8436, -27.7606) (-166.8096, -27.7442) (-166.7755, -27.7279) (-166.7413, -27.7118) (-166.7069, -27.6958) (-166.6724, -27.68) (-166.6377, -27.6643) (-166.603, -27.6488) (-166.575, -27.6365) (-166.554, -27.6273) (-166.54, -27.6212) (-166.533, -27.6182) knots 0 0 0 0 0 0 0.01428571 0.02857143 0.04285714 0.05714286 0.07142857 0.08571429 0.1 0.11428571 0.12857143 0.14285714 0.15714286 0.17142857 0.18571429 0.2 0.21428571 0.22857143 0.24285714 0.25714286 0.27142857 0.28571429 0.3 0.31428571 0.32857143 0.34285714 0.35714286 0.37142857 0.38571429 0.4 0.41428571 0.42857143 0.44285714 0.45714286 0.47142857 0.48571429 0.5 0.51428571 0.52857143 0.54285714 0.55714286 0.57142857 0.58571429 0.6 0.61428571 0.62857143 0.64285714 0.65714286 0.67142857 0.68571429 0.7 0.71428571 0.72857143 0.74285714 0.75714286 0.77142857 0.78571429 0.8 0.81428571 0.82857143 0.84285714 0.85714286 0.87142857 0.88571429 0.9 0.91428571 0.92857143 0.94285714 0.95714286 0.97142857 0.98571429 1 1 1 1 1 1
  line L27 (-168.5683, -29.0655) -> (-168.7871, -29.4375)
  arc A54 (-169.4538, -29.6249) -> (-168.7871, -29.4375) centre (-169.218, -29.184) ccw
  arc A55 (-169.4538, -29.6249) -> (-170.1793, -29.2685) centre (-175, -40) ccw
  arc A56 (-170.4385, -28.6263) -> (-170.1793, -29.2685) centre (-169.9744, -28.8125) ccw
  line L28 (-170.4385, -28.6263) -> (-170.2778, -28.2258)
  spline S28 degree 5 poles (-170.2778, -28.2258) (-170.2753, -28.2195) (-170.2704, -28.2068) (-170.2636, -28.1876) (-170.2556, -28.1617) (-170.2469, -28.1289) (-170.2392, -28.0957) (-170.2321, -28.0622) (-170.2254, -28.0287) (-170.2188, -27.995) (-170.2126, -27.9613) (-170.2066, -27.9275) (-170.201, -27.8935) (-170.1959, -27.8594) (-170.1913, -27.8251) (-170.1872, -27.7907) (-170.1834, -27.7562) (-170.18, -27.7215) (-170.1769, -27.6868) (-170.174, -27.652) (-170.1714, -27.6172) (-170.1691, -27.5822) (-170.1671, -27.5472) (-170.1654, -27.512) (-170.1641, -27.4768) (-170.163, -27.4415) (-170.1622, -27.4062) (-170.1616, -27.3708) (-170.1613, -27.3353) (-170.1613, -27.2997) (-170.1616, -27.2641) (-170.162, -27.2284) (-170.1628, -27.1927) (-170.1638, -27.1569) (-170.165, -27.121) (-170.1665, -27.0851) (-170.1682, -27.0492) (-170.1702, -27.0131) (-170.1724, -26.9771) (-170.1749, -26.941) (-170.1775, -26.9048) (-170.1804, -26.8686) (-170.1836, -26.8324) (-170.1869, -26.7961) (-170.1905, -26.7598) (-170.1943, -26.7234) (-170.1983, -26.687) (-170.2026, -26.6505) (-170.2071, -26.6141) (-170.2117, -26.5776) (-170.2166, -26.541) (-170.2218, -26.5044) (-170.2271, -26.4678) (-170.2326, -26.4312) (-170.2384, -26.3945) (-170.2443, -26.3578) (-170.2505, -26.321) (-170.2569, -26.2843) (-170.2634, -26.2475) (-170.2702, -26.2107) (-170.2772, -26.1739) (-170.2844, -26.137) (-170.2918, -26.1001) (-170.2993, -26.0632) (-170.3071, -26.0263) (-170.3151, -25.9894) (-170.3233, -25.9524) (-170.3317, -25.9154) (-170.3402, -25.8785) (-170.349, -25.8414) (-170.358, -25.8044) (-170.3653, -25.7748) (-170.3709, -25.7526) (-170.3746, -25.7377) (-170.3765, -25.7303) knots 0 0 0 0 0 0 0.01428571 0.02857143 0.04285714 0.05714286 0.07142857 0.08571429 0.1 0.11428571 0.12857143 0.14285714 0.15714286 0.17142857 0.18571429 0.2 0.21428571 0.22857143 0.24285714 0.25714286 0.27142857 0.28571429 0.3 0.31428571 0.32857143 0.34285714 0.35714286 0.37142857 0.38571429 0.4 0.41428571 0.42857143 0.44285714 0.45714286 0.47142857 0.48571429 0.5 0.51428571 0.52857143 0.54285714 0.55714286 0.57142857 0.58571429 0.6 0.61428571 0.62857143 0.64285714 0.65714286 0.67142857 0.68571429 0.7 0.71428571 0.72857143 0.74285714 0.75714286 0.77142857 0.78571429 0.8 0.81428571 0.82857143 0.84285714 0.85714286 0.87142857 0.88571429 0.9 0.91428571 0.92857143 0.94285714 0.95714286 0.97142857 0.98571429 1 1 1 1 1 1
  arc A57 (-170.3765, -25.7303) -> (-171.2784, -25.469) centre (-175, -40) ccw
  spline S29 degree 5 poles (-172.696, -27.5251) (-172.6947, -27.5185) (-172.6921, -27.5051) (-172.6876, -27.4853) (-172.6805, -27.4591) (-172.6703, -27.4267) (-172.6591, -27.3945) (-172.6472, -27.3625) (-172.6349, -27.3305) (-172.6225, -27.2986) (-172.6097, -27.2667) (-172.5967, -27.2349) (-172.5833, -27.2033) (-172.5693, -27.1717) (-172.5549, -27.1403) (-172.54, -27.109) (-172.5247, -27.0778) (-172.509, -27.0467) (-172.4931, -27.0157) (-172.4769, -26.9848) (-172.4605, -26.9539) (-172.4437, -26.9231) (-172.4267, -26.8924) (-172.4094, -26.8619) (-172.3917, -26.8314) (-172.3738, -26.801) (-172.3555, -26.7707) (-172.3371, -26.7404) (-172.3183, -26.7103) (-172.2993, -26.6802) (-172.2801, -26.6502) (-172.2606, -26.6203) (-172.2409, -26.5905) (-172.2209, -26.5608) (-172.2007, -26.5312) (-172.1802, -26.5016) (-172.1595, -26.4722) (-172.1386, -26.4428) (-172.1175, -26.4135) (-172.0961, -26.3843) (-172.0745, -26.3552) (-172.0527, -26.3261) (-172.0307, -26.2972) (-172.0085, -26.2683) (-171.986, -26.2395) (-171.9633, -26.2108) (-171.9405, -26.1822) (-171.9174, -26.1537) (-171.8941, -26.1252) (-171.8706, -26.0969) (-171.847, -26.0686) (-171.8231, -26.0404) (-171.799, -26.0123) (-171.7747, -25.9843) (-171.7503, -25.9564) (-171.7256, -25.9286) (-171.7008, -25.9008) (-171.6757, -25.8732) (-171.6505, -25.8456) (-171.6251, -25.8181) (-171.5995, -25.7907) (-171.5737, -25.7634) (-171.5478, -25.7362) (-171.5216, -25.7091) (-171.4953, -25.682) (-171.4688, -25.6551) (-171.4422, -25.6282) (-171.4153, -25.6015) (-171.3883, -25.5748) (-171.3611, -25.5482) (-171.3337, -25.5217) (-171.3117, -25.5006) (-171.2951, -25.4848) (-171.284, -25.4743) (-171.2784, -25.469) knots 0 0 0 0 0 0 0.01428571 0.02857143 0.04285714 0.05714286 0.07142857 0.08571429 0.1 0.11428571 0.12857143 0.14285714 0.15714286 0.17142857 0.18571429 0.2 0.21428571 0.22857143 0.24285714 0.25714286 0.27142857 0.28571429 0.3 0.31428571 0.32857143 0.34285714 0.35714286 0.37142857 0.38571429 0.4 0.41428571 0.42857143 0.44285714 0.45714286 0.47142857 0.48571429 0.5 0.51428571 0.52857143 0.54285714 0.55714286 0.57142857 0.58571429 0.6 0.61428571 0.62857143 0.64285714 0.65714286 0.67142857 0.68571429 0.7 0.71428571 0.72857143 0.74285714 0.75714286 0.77142857 0.78571429 0.8 0.81428571 0.82857143 0.84285714 0.85714286 0.87142857 0.88571429 0.9 0.91428571 0.92857143 0.94285714 0.95714286 0.97142857 0.98571429 1 1 1 1 1 1
  line L29 (-172.696, -27.5251) -> (-172.7744, -27.9495)
  arc A58 (-173.3367, -28.3537) -> (-172.7744, -27.9495) centre (-173.266, -27.8587) ccw
  arc A59 (-173.3367, -28.3537) -> (-174.1404, -28.2669) centre (-175, -40) ccw
  arc A60 (-174.6036, -27.7521) -> (-174.1404, -28.2669) centre (-174.1038, -27.7683) ccw
  line L30 (-174.6036, -27.7521) -> (-174.5896, -27.3208)
  spline S30 degree 5 poles (-174.5896, -27.3208) (-174.5894, -27.314) (-174.5891, -27.3004) (-174.5893, -27.2801) (-174.5906, -27.253) (-174.5937, -27.2191) (-174.5978, -27.1853) (-174.6026, -27.1515) (-174.6077, -27.1176) (-174.6131, -27.0838) (-174.6187, -27.0499) (-174.6247, -27.0161) (-174.6311, -26.9823) (-174.638, -26.9485) (-174.6454, -26.9147) (-174.6533, -26.8809) (-174.6615, -26.8472) (-174.6702, -26.8135) (-174.6791, -26.7798) (-174.6883, -26.7461) (-174.6978, -26.7125) (-174.7076, -26.6788) (-174.7177, -26.6452) (-174.7281, -26.6116) (-174.7389, -26.5781) (-174.7499, -26.5446) (-174.7613, -26.511) (-174.7729, -26.4776) (-174.7847, -26.4441) (-174.7969, -26.4107) (-174.8093, -26.3773) (-174.8219, -26.344) (-174.8349, -26.3106) (-174.848, -26.2773) (-174.8615, -26.2441) (-174.8751, -26.2108) (-174.8891, -26.1776) (-174.9032, -26.1445) (-174.9177, -26.1113) (-174.9323, -26.0782) (-174.9472, -26.0452) (-174.9623, -26.0121) (-174.9776, -25.9792) (-174.9932, -25.9462) (-175.009, -25.9133) (-175.025, -25.8804) (-175.0412, -25.8476) (-175.0577, -25.8148) (-175.0744, -25.7821) (-175.0913, -25.7493) (-175.1084, -25.7167) (-175.1257, -25.684) (-175.1432, -25.6515) (-175.1609, -25.6189) (-175.1789, -25.5864) (-175.197, -25.554) (-175.2154, -25.5216) (-175.2339, -25.4892) (-175.2527, -25.4569) (-175.2717, -25.4246) (-175.2908, -25.3924) (-175.3102, -25.3602) (-175.3297, -25.3281) (-175.3495, -25.296) (-175.3694, -25.264) (-175.3896, -25.232) (-175.4099, -25.2001) (-175.4304, -25.1682) (-175.4511, -25.1364) (-175.472, -25.1046) (-175.4931, -25.0729) (-175.5101, -25.0475) (-175.523, -25.0285) (-175.5316, -25.0159) (-175.5359, -25.0096) knots 0 0 0 0 0 0 0.01428571 0.02857143 0.04285714 0.05714286 0.07142857 0.08571429 0.1 0.11428571 0.12857143 0.14285714 0.15714286 0.17142857 0.18571429 0.2 0.21428571 0.22857143 0.24285714 0.25714286 0.27142857 0.28571429 0.3 0.31428571 0.32857143 0.34285714 0.35714286 0.37142857 0.38571429 0.4 0.41428571 0.42857143 0.44285714 0.45714286 0.47142857 0.48571429 0.5 0.51428571 0.52857143 0.54285714 0.55714286 0.57142857 0.58571429 0.6 0.61428571 0.62857143 0.64285714 0.65714286 0.67142857 0.68571429 0.7 0.71428571 0.72857143 0.74285714 0.75714286 0.77142857 0.78571429 0.8 0.81428571 0.82857143 0.84285714 0.85714286 0.87142857 0.88571429 0.9 0.91428571 0.92857143 0.94285714 0.95714286 0.97142857 0.98571429 1 1 1 1 1 1
  arc A61 (-175.5359, -25.0096) -> (-176.4728, -25.0725) centre (-175, -40) ccw
  spline S31 degree 5 poles (-177.1016, -27.4894) (-177.1027, -27.4827) (-177.1048, -27.4693) (-177.1073, -27.4491) (-177.1097, -27.4221) (-177.1111, -27.3881) (-177.1116, -27.3541) (-177.1113, -27.3199) (-177.1108, -27.2857) (-177.11, -27.2514) (-177.1089, -27.2171) (-177.1076, -27.1828) (-177.1057, -27.1484) (-177.1034, -27.114) (-177.1006, -27.0795) (-177.0973, -27.045) (-177.0936, -27.0105) (-177.0896, -26.9759) (-177.0852, -26.9413) (-177.0806, -26.9067) (-177.0757, -26.8721) (-177.0705, -26.8375) (-177.0649, -26.8028) (-177.0591, -26.7681) (-177.0529, -26.7334) (-177.0465, -26.6987) (-177.0397, -26.664) (-177.0327, -26.6293) (-177.0254, -26.5946) (-177.0178, -26.5598) (-177.01, -26.5251) (-177.0019, -26.4903) (-176.9936, -26.4556) (-176.985, -26.4208) (-176.9761, -26.386) (-176.967, -26.3513) (-176.9576, -26.3165) (-176.948, -26.2817) (-176.9382, -26.247) (-176.9281, -26.2122) (-176.9178, -26.1775) (-176.9072, -26.1427) (-176.8964, -26.108) (-176.8854, -26.0733) (-176.8741, -26.0385) (-176.8627, -26.0038) (-176.8509, -25.9691) (-176.839, -25.9344) (-176.8269, -25.8997) (-176.8145, -25.865) (-176.8019, -25.8304) (-176.7891, -25.7957) (-176.7761, -25.7611) (-176.7629, -25.7265) (-176.7494, -25.6919) (-176.7358, -25.6573) (-176.7219, -25.6227) (-176.7079, -25.5882) (-176.6936, -25.5536) (-176.6791, -25.5191) (-176.6644, -25.4846) (-176.6496, -25.4501) (-176.6345, -25.4157) (-176.6192, -25.3812) (-176.6037, -25.3468) (-176.588, -25.3125) (-176.5722, -25.2781) (-176.5561, -25.2438) (-176.5398, -25.2094) (-176.5234, -25.1752) (-176.5067, -25.1409) (-176.4932, -25.1135) (-176.483, -25.093) (-176.4762, -25.0793) (-176.4728, -25.0725) knots 0 0 0 0 0 0 0.01428571 0.02857143 0.04285714 0.05714286 0.07142857 0.08571429 0.1 0.11428571 0.12857143 0.14285714 0.15714286 0.17142857 0.18571429 0.2 0.21428571 0.22857143 0.24285714 0.25714286 0.27142857 0.28571429 0.3 0.31428571 0.32857143 0.34285714 0.35714286 0.37142857 0.38571429 0.4 0.41428571 0.42857143 0.44285714 0.45714286 0.47142857 0.48571429 0.5 0.51428571 0.52857143 0.54285714 0.55714286 0.57142857 0.58571429 0.6 0.61428571 0.62857143 0.64285714 0.65714286 0.67142857 0.68571429 0.7 0.71428571 0.72857143 0.74285714 0.75714286 0.77142857 0.78571429 0.8 0.81428571 0.82857143 0.84285714 0.85714286 0.87142857 0.88571429 0.9 0.91428571 0.92857143 0.94285714 0.95714286 0.97142857 0.98571429 1 1 1 1 1 1
  line L31 (-177.1016, -27.4894) -> (-177.0301, -27.915)
  arc A62 (-177.4203, -28.4872) -> (-177.0301, -27.915) centre (-177.5232, -27.9979) ccw
  arc A63 (-177.4203, -28.4872) -> (-178.2052, -28.6805) centre (-175, -40) ccw
  arc A64 (-178.8165, -28.3552) -> (-178.2052, -28.6805) centre (-178.3414, -28.1994) ccw
  line L32 (-178.8165, -28.3552) -> (-178.9509, -27.9451)